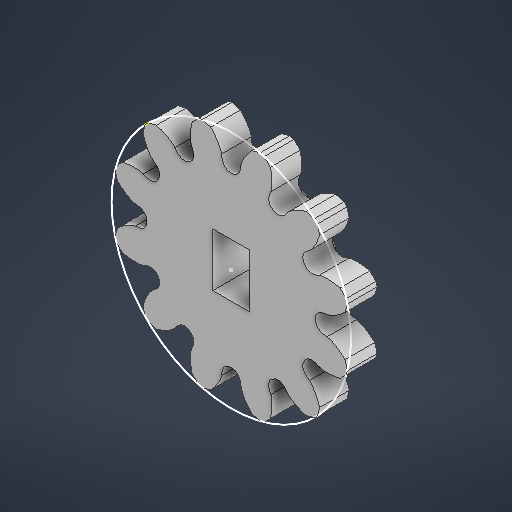
# Autodesk Inventor part: DoorPinion
Saved by Autodesk Inventor 2026.1 (Build 301233000, 233)
## iProperties
Created: 2026-02-25
Part Number: DoorPinion
Material: Generic
Document SubType Name: Sheet Metal
Designer: ba2032
Density: 1 g/cm^3
Appearance: Default
Sheet Metal Rule: Default
Author: ba2032
Autodesk Inventor part; units mm, degrees
ref_plane "YZ Plane" through (0, 0, 0) normal (1, 0, 0) x (0, 1, 0)
ref_plane "XZ Plane" through (0, 0, 0) normal (0, 1, 0) x (-1, 0, 0)
ref_plane "XY Plane" through (0, 0, 0) normal (0, 0, 1) x (1, 0, 0)
sketch "Sketch1" plane through (0, 0, 0) normal (0, 0, 1) x (1, 0, 0)
  spline S0 degree 3 poles (-61.7215, 300.6455) (-59.6627, 298.7497) (-55.5452, 294.958) (-49.7389, 288.8881) (-44.2406, 282.5405) (-39.1259, 275.8781) (-35.2296, 270.0612) (-32.3803, 265.2431) (-30.394, 261.5443) (-28.575, 257.759) (-26.9725, 253.8799) (-25.5655, 249.9169) (-24.9973, 247.1751) (-24.7133, 245.8047) knots 0 0 0 0 0.839437 1.67888 2.518311 3.357718 4.197088 4.61683 5.036567 5.456294 5.876005 6.295675 6.715083 6.715083 6.715083 6.715083
  spline S1 degree 3 poles (-24.7133, 245.8047) (-24.5917, 243.9908) (-24.4093, 241.2697) (-23.872, 237.6708) (-23.246, 235.0152) (-22.4945, 232.3916) (-21.4907, 229.8531) (-20.3061, 227.3947) (-18.8736, 225.0688) (-17.186, 222.9208) (-15.2479, 220.9937) (-13.0645, 219.3517) (-10.6906, 217.9952) (-8.133, 217.0268) (-5.4577, 216.4349) (-2.7248, 216.3531) (0, 216.3899) (2.7248, 216.3531) (5.4577, 216.4349) (8.133, 217.0268) (10.6906, 217.9952) (13.0645, 219.3517) (15.2479, 220.9937) (17.186, 222.9208) (18.8736, 225.0688) (20.3061, 227.3947) (21.4907, 229.8531) (22.4945, 232.3916) (23.246, 235.0152) (23.872, 237.6708) (24.4093, 241.2697) (24.5917, 243.9908) (24.7133, 245.8047) knots 0 0 0 0 0.545156 0.817799 1.090469 1.363152 1.635764 1.908322 2.180933 2.453514 2.726009 2.99841 3.270864 3.543393 3.816007 4.088487 4.361176 4.633865 4.906345 5.178959 5.451488 5.723942 5.996343 6.268838 6.54142 6.814031 7.086588 7.3592 7.631883 7.904554 8.177197 8.722353 8.722353 8.722353 8.722353
  spline S2 degree 3 poles (24.7133, 245.8047) (24.9973, 247.1751) (25.5655, 249.9169) (26.9725, 253.8799) (28.575, 257.759) (30.394, 261.5443) (32.3803, 265.2431) (35.2296, 270.0612) (39.1259, 275.8781) (44.2406, 282.5405) (49.7389, 288.8881) (55.5452, 294.958) (59.6627, 298.7497) (61.7215, 300.6455) knots 0 0 0 0 0.419408 0.839079 1.258789 1.678516 2.098253 2.517995 3.357365 4.196772 5.036203 5.875647 6.715083 6.715083 6.715083 6.715083
  circle A0 centre (0, 0) radius 216.3776 construction
  circle A1 centre (0, 0) radius 246.9254 construction
  circle A2 centre (0, 0) radius 262.7726 construction
  circle A3 centre (0, 0) radius 306.9157
  point P0 (-55.6069, 294.8943)
  point P1 (-49.7902, 288.8418)
  point P2 (-44.3045, 282.4879)
  point P3 (-39.199, 275.825)
  point P4 (-34.5398, 268.8432)
  point P5 (-32.4054, 265.2289)
  point P6 (-30.4219, 261.5298)
  point P7 (-28.6111, 257.7432)
  point P8 (-27.005, 253.8656)
  point P9 (-25.6577, 249.891)
  point P10 (-24.2505, 240.3728)
  point P11 (-23.8348, 237.6782)
  point P12 (-23.2251, 235.0206)
  point P13 (-22.4523, 232.4055)
  point P14 (-21.4605, 229.8662)
  point P15 (-20.2649, 227.4169)
  point P16 (-18.831, 225.0983)
  point P17 (-17.144, 222.9573)
  point P18 (-15.2068, 221.0409)
  point P19 (-13.0329, 219.3994)
  point P20 (-10.6603, 218.06)
  point P21 (-8.1136, 217.0896)
  point P22 (-5.4477, 216.5198)
  point P23 (-2.7269, 216.3729)
  point P24 (0, 216.3776)
  point P25 (2.7269, 216.3729)
  point P26 (5.4477, 216.5198)
  point P27 (8.1136, 217.0896)
  point P28 (10.6603, 218.06)
  point P29 (13.0329, 219.3994)
  point P30 (15.2068, 221.0409)
  point P31 (17.144, 222.9573)
  point P32 (18.831, 225.0983)
  point P33 (20.2649, 227.4169)
  point P34 (21.4605, 229.8662)
  point P35 (22.4523, 232.4055)
  point P36 (23.2251, 235.0206)
  point P37 (23.8348, 237.6782)
  point P38 (24.2505, 240.3728)
  point P39 (25.6577, 249.891)
  point P40 (27.005, 253.8656)
  point P41 (28.6111, 257.7432)
  point P42 (30.4219, 261.5298)
  point P43 (32.4054, 265.2289)
  point P44 (34.5398, 268.8432)
  point P45 (39.199, 275.825)
  point P46 (44.3045, 282.4879)
  point P47 (49.7902, 288.8418)
  point P48 (55.6069, 294.8943)
  constraints: 4 centre point, 2 point on circle, 113 other
extrude "Extrusion1" add sketch "Sketch1" against normal blind 76.2
extrude "Extrusion2" cut sketch "Sketch1" against normal blind 76.2 contours A3 S2 S1 S0 picked at (1.2398, 274.8749)
pattern_circular "Circular Pattern1" count 12 over 360 about axis through (0, 0, -10) along (0, 0, 1) of "Extrusion2"
sketch "Sketch2" plane through (0, 0, 0) normal (0, 0, 1) x (1, 0, 0)
  line L0 (46.99, -68.58) -> (-46.99, -68.58)
  line L1 (-46.99, -68.58) -> (-46.99, 68.58)
  line L2 (-46.99, 68.58) -> (46.99, 68.58)
  line L3 (46.99, 68.58) -> (46.99, -68.58)
  line L4 (46.99, -68.58) -> (-46.99, 68.58) construction
  line L5 (-46.99, -68.58) -> (46.99, 68.58) construction
  point P0 (0, 0)
  dimension "d7" = 93.98
  dimension "d8" = 137.16
  constraints: 12 end point, 2 midpoint, 2 parallel, 1 horizontal, 1 perpendicular
  measures "d7" distance of L1.end L2.end
  measures "d8" distance of L0.end L1.end
extrude "Extrusion3" cut sketch "Sketch2" against normal blind 76.2
sketch "Sketch3" plane through (0, 0, -76.2) normal (0, 0, -1) x (-1, 0, 0)
  circle A0 centre (0, 0) radius 152.4
  dimension "d11" = 304.8
  constraints: 1 centre point, 1 coincident
  measures "d11" diameter of A0
extrude "Extrusion4" add sketch "Sketch3" along normal blind 50.8
sketch "Sketch4" plane through (0, 0, -127) normal (0, 0, -1) x (-1, 0, 0)
  line L0 (46.99, 68.58) -> (-46.99, 68.58)
  line L1 (-46.99, 68.58) -> (-46.99, -68.58)
  line L2 (-46.99, -68.58) -> (46.99, -68.58)
  line L3 (46.99, -68.58) -> (46.99, 68.58)
  line L4 (46.99, 68.58) -> (-46.99, -68.58) construction
  line L5 (-46.99, 68.58) -> (46.99, -68.58) construction
  point P0 (0, 0)
  dimension "d14" = 93.98
  dimension "d15" = 137.16
  constraints: 12 end point, 2 midpoint, 2 parallel, 1 horizontal, 1 perpendicular
  measures "d14" distance of L2.end L1.end
  measures "d15" distance of L1.end L0.end
extrude "Extrusion5" cut sketch "Sketch4" against normal blind 50.8
chamfer "Chamfer1" distance 12.7 angle 45 1 edges at (203.7751, 229.5059, -38.1)
chamfer "Chamfer2" distance 12.7 angle 45 1 edges at (96.8703, 291.2274, -38.1)
chamfer "Chamfer3" distance 12.7 angle 45 1 edges at (61.7215, 300.6455, -38.1)
chamfer "Chamfer4" distance 12.7 angle 45 1 edges at (-61.7215, 300.6455, -38.1)
chamfer "Chamfer5" distance 12.7 angle 45 1 edges at (-96.8703, 291.2274, -38.1)
chamfer "Chamfer6" distance 12.7 angle 45 1 edges at (229.5059, 203.7751, -38.1)
chamfer "Chamfer7" distance 12.7 angle 45 1 edges at (291.2274, 96.8703, -38.1)
chamfer "Chamfer8" distance 12.7 angle 45 1 edges at (-203.7751, 229.5059, -38.1)
chamfer "Chamfer9" distance 12.7 angle 45 1 edges at (-291.2274, 96.8703, -38.1)
chamfer "Chamfer10" distance 12.7 angle 45 1 edges at (300.6455, -61.7215, -38.1)
chamfer "Chamfer11" distance 12.7 angle 45 1 edges at (291.2274, -96.8703, -38.1)
chamfer "Chamfer12" distance 12.7 angle 45 1 edges at (229.5059, -203.7751, -38.1)
chamfer "Chamfer13" distance 12.7 angle 45 1 edges at (96.8703, -291.2274, -38.1)
chamfer "Chamfer14" distance 12.7 angle 45 1 edges at (-61.7215, -300.6455, -38.1)
chamfer "Chamfer15" distance 12.7 angle 45 1 edges at (300.6455, 61.7215, -38.1)
chamfer "Chamfer16" distance 12.7 angle 45 1 edges at (61.7215, -300.6455, -38.1)
chamfer "Chamfer17" distance 12.7 angle 45 1 edges at (-96.8703, -291.2274, -38.1)
chamfer "Chamfer18" distance 12.7 angle 45 1 edges at (-203.7751, -229.5059, -38.1)
chamfer "Chamfer19" distance 12.7 angle 45 1 edges at (-229.5059, -203.7751, -38.1)
chamfer "Chamfer20" distance 12.7 angle 45 1 edges at (-291.2274, -96.8703, -38.1)
chamfer "Chamfer21" distance 12.7 angle 45 1 edges at (-300.6455, -61.7215, -38.1)
chamfer "Chamfer22" distance 12.7 angle 45 1 edges at (203.7751, -229.5059, -38.1)
chamfer "Chamfer23" distance 12.7 angle 45 1 edges at (-300.6455, 61.7215, -38.1)
chamfer "Chamfer24" distance 12.7 angle 45 1 edges at (-229.5059, 203.7751, -38.1)
scale "Scale1" factors (0.03937, 0.03937, 0.03937) then translate (0, 0, 0) bodies 1
sketch "Sketch5" plane through (0, 9.0981, 0) normal (0, 0, 1) x (0.9977601, 0.0668934, 0)
  point P0 (-0.6086, -9.0777)
sketch "Sketch6" plane through (0, 9.0981, 0) normal (0, 0, 1) x (0.9977601, 0.0668934, 0)
  point P0 (-0.6086, -9.0777)
sketch "Sketch7" plane through (0, 9.0981, 0) normal (0, 0, 1) x (0.9977601, 0.0668934, 0)
  arc A0 (-8.3977, 0.1601) -> (-8.7239, -0.1252) centre (-0.6086, -9.0777) ccw projected
  circle A1 centre (-0.6086, -9.0777) radius 12.0833
  constraints: 1 coincident, 3 other
equation "\"Module\" = 40.42655"
equation "\"PressureAngle\" = 20deg"
equation "\"UnitProfileClearance\" = 0.25"
equation "\"UnitRoundRadius\" = 0.35"
equation "\"HeadDiameter\" = 613.83143"
equation "\"RootDiameter\" = 432.7553"
equation "\"BaseDiameter\" = 493.85087"
equation "\"PitchDiameter\" = 525.54512"
equation "\"FaceWidth\" = 50.8"
equation "\"HelixAngle\" = 0"
equation "\"UnitCorrection\" = 0.102365"
equation "\"UnitAddendumModification\" = 0.01043"
equation "\"CircularPitch\" = 127.00375"
equation "\"UnitBacklashShift\" = 0"
equation "\"TotalToolShift\" = 4.13827"
equation "\"IsInternal\" = 0"
equation "\"BendRadius\" = Thickness"
equation "\"BendReliefWidth\" = Thickness"
equation "\"BendReliefDepth\" = 0.5 * Thickness"
equation "\"CornerReliefSize\" = 4 * Thickness"
equation "\"MinimumRemnant\" = 2 * Thickness"
equation "\"TransitionRadius\" = BendRadius"
equation "\"JacobiRadiusSize\" = BendRadius"
equation "\"GapSize\" = Thickness"
equation "\"Thickness\" = 3.048"
body "Solid1"
